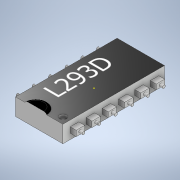
# Autodesk Inventor part: drive motor
Saved by Autodesk Inventor 2021 (Build 250183000, 183)
## iProperties
Created: 2021-07-29
Part Number: drive motor
Material: Generic
Document SubType Name: Modeling
Designer: Dell
Density: 1 g/cm^3
Appearance: Default
Author: Dell
Autodesk Inventor part; units mm, degrees
ref_plane "YZ Plane" through (0, 0, 0) normal (1, 0, 0) x (0, 1, 0)
ref_plane "XZ Plane" through (0, 0, 0) normal (0, 1, 0) x (-1, 0, 0)
ref_plane "XY Plane" through (0, 0, 0) normal (0, 0, 1) x (1, 0, 0)
sketch "Sketch1" plane through (0, 0, 0) normal (0, 1, 0) x (-1, 0, 0)
  line L0 (-9.2195, 27.5122) -> (18.7805, 27.5122)
  line L1 (18.7805, 27.5122) -> (18.7805, -32.4878)
  line L2 (18.7805, -32.4878) -> (-9.2195, -32.4878)
  line L3 (-9.2195, -32.4878) -> (-9.2195, 27.5122)
  point P0 (0, 0)
  dimension "d0" = 60
  dimension "d1" = 28
  constraints: 8 end point, 2 parallel, 1 horizontal, 1 perpendicular
  measures "d0" distance of L0.end L1.end
  measures "d1" distance of L0.start L0.end
extrude "Extrusion1" add sketch "Sketch1" along normal blind 10
sketch "Sketch2" plane through (9.2195, 0, 27.5122) normal (1, 0, 0) x (0, 0, -1)
  line L0 (60, 10) -> (0, 10) projected
  line L1 (60, 0) -> (0, 0) projected
  line L2 (4.3635, 6.5) -> (9.3635, 6.5)
  line L3 (9.3635, 6.5) -> (9.3635, 3.2102)
  line L4 (9.3635, 3.2102) -> (4.3635, 3.2102)
  line L5 (4.3635, 3.2102) -> (4.3635, 6.5)
  line L6 (13.6667, 6.5) -> (18.6667, 6.5)
  line L7 (18.6667, 6.5) -> (18.6667, 3.2102)
  line L8 (18.6667, 3.2102) -> (13.6667, 3.2102)
  line L9 (13.6667, 3.2102) -> (13.6667, 6.5)
  line L10 (23.1882, 6.5) -> (28.1882, 6.5)
  line L11 (28.1882, 6.5) -> (28.1882, 3.5)
  line L12 (28.1882, 3.5) -> (23.1882, 3.5)
  line L13 (23.1882, 3.5) -> (23.1882, 6.5)
  line L14 (32.8844, 6.5) -> (37.8844, 6.5)
  line L15 (37.8844, 6.5) -> (37.8844, 3.5)
  line L16 (37.8844, 3.5) -> (32.8844, 3.5)
  line L17 (32.8844, 3.5) -> (32.8844, 6.5)
  line L18 (42.406, 6.5) -> (47.406, 6.5)
  line L19 (47.406, 6.5) -> (47.406, 3.5)
  line L20 (47.406, 3.5) -> (42.406, 3.5)
  line L21 (42.406, 3.5) -> (42.406, 6.5)
  line L22 (51.5781, 6.5) -> (56.5781, 6.5)
  line L23 (56.5781, 6.5) -> (56.5781, 3.5)
  line L24 (56.5781, 3.5) -> (51.5781, 3.5)
  line L25 (51.5781, 3.5) -> (51.5781, 6.5)
  point P0 (27.5122, 0)
  point P1 (4.3635, 10)
  point P2 (4.3635, 0)
  point P3 (4.3635, 3.5)
  dimension "d4" = 10
  dimension "d5" = 3
  dimension "d6" = 3.5
  dimension "d7" = 3.5
  dimension "d8" = 5
  dimension "d9" = 5
  dimension "d10" = 5
  dimension "d11" = 5
  dimension "d12" = 5
  dimension "d13" = 5
  constraints: 48 end point, 12 parallel, 11 point on line, 6 horizontal, 6 perpendicular
  measures "d4" distance of point (4.364, 0) point (4.364, 10)
  measures "d5" distance of point (4.364, 3.5) L2.start
  measures "d6" distance of point (4.364, 0) point (4.364, 3.5)
  measures "d7" distance of point (4.364, 10) L2.start
  measures "d8" distance of L6.start L6.end
  measures "d9" distance of L2.start L2.end
  measures "d10" distance of L10.start L10.end
  measures "d11" distance of L14.start L14.end
  measures "d12" distance of L18.start L18.end
  measures "d13" distance of L22.start L22.end
extrude "Extrusion2" add sketch "Sketch2" along normal blind 3.5
sketch "Sketch3" plane through (-18.7805, 0, -32.4878) normal (-1, 0, 0) x (0, 0, 1)
  line L0 (3.4219, 6.5) -> (3.4219, 3.5) projected
  line L1 (8.4219, 3.5) -> (3.4219, 3.5) projected
  line L2 (3.4219, 6.5) -> (8.4219, 6.5)
  line L3 (8.4219, 6.5) -> (8.4219, 3.5)
  line L4 (8.4219, 3.5) -> (3.4219, 3.5)
  line L5 (3.4219, 3.5) -> (3.4219, 6.5)
  line L6 (12.594, 3.5) -> (12.594, 6.5) projected
  line L7 (17.594, 6.5) -> (17.594, 3.5) projected
  line L8 (12.594, 6.5) -> (17.594, 6.5)
  line L9 (17.594, 6.5) -> (17.594, 3.5)
  line L10 (17.594, 3.5) -> (12.594, 3.5)
  line L11 (12.594, 3.5) -> (12.594, 6.5)
  line L12 (22.1156, 6.5) -> (27.1156, 6.5) projected
  line L13 (27.1156, 6.5) -> (27.1156, 3.5) projected
  line L14 (22.1156, 6.5) -> (27.1156, 6.5)
  line L15 (27.1156, 6.5) -> (27.1156, 3.5)
  line L16 (27.1156, 3.5) -> (22.1156, 3.5)
  line L17 (22.1156, 3.5) -> (22.1156, 6.5)
  line L18 (31.8118, 6.5) -> (31.8118, 3.5) projected
  line L19 (36.8118, 6.5) -> (36.8118, 3.5) projected
  line L20 (31.8118, 6.5) -> (36.8118, 6.5)
  line L21 (36.8118, 6.5) -> (36.8118, 3.5)
  line L22 (36.8118, 3.5) -> (31.8118, 3.5)
  line L23 (31.8118, 3.5) -> (31.8118, 6.5)
  line L24 (41.3333, 3.2102) -> (41.3333, 6.5) projected
  line L25 (46.3333, 3.2102) -> (41.3333, 3.2102) projected
  line L26 (41.3333, 6.5) -> (46.3333, 6.5)
  line L27 (46.3333, 6.5) -> (46.3333, 3.2102)
  line L28 (46.3333, 3.2102) -> (41.3333, 3.2102)
  line L29 (41.3333, 3.2102) -> (41.3333, 6.5)
  line L30 (50.6365, 3.2102) -> (50.6365, 6.5) projected
  line L31 (55.6365, 3.2102) -> (50.6365, 3.2102) projected
  line L32 (50.6365, 6.5) -> (55.6365, 6.5)
  line L33 (55.6365, 6.5) -> (55.6365, 3.2102)
  line L34 (55.6365, 3.2102) -> (50.6365, 3.2102)
  line L35 (50.6365, 3.2102) -> (50.6365, 6.5)
  point P0 (32.4878, 0)
  constraints: 48 end point, 12 parallel, 6 horizontal, 6 perpendicular
extrude "Extrusion3" add sketch "Sketch3" along normal blind 3.5
sketch "Sketch4" plane through (-22.2805, 0, -32.4878) normal (-1, 0, 0) x (0, 0, 1)
  circle A0 centre (5.9219, 4.87) radius 0.85
  circle A1 centre (15.1045, 4.87) radius 0.85
  circle A2 centre (24.4513, 4.87) radius 0.85
  circle A3 centre (34.1912, 4.87) radius 0.85
  circle A4 centre (43.8874, 4.8551) radius 0.85
  circle A5 centre (53.3216, 4.8551) radius 0.85
  point P0 (32.4878, 0)
  dimension "d18" = 1.7
  dimension "d19" = 1.7
  dimension "d20" = 1.7
  dimension "d21" = 1.7
  dimension "d22" = 1.7
  dimension "d23" = 1.7
  constraints: 6 centre point
  measures "d18" diameter of A0
  measures "d19" diameter of A1
  measures "d20" diameter of A2
  measures "d21" diameter of A3
  measures "d22" diameter of A4
  measures "d23" diameter of A5
extrude "Extrusion4" add sketch "Sketch4" along normal blind 2
sketch "Sketch5" plane through (9.2195, 0, 27.5122) normal (1, 0, 0) x (0, 0, -1)
  circle A0 centre (6.6784, 4.8551) radius 0.85 projected
  circle A1 centre (6.6784, 4.8551) radius 0.85
  circle A2 centre (16.1126, 4.8551) radius 0.85 projected
  circle A3 centre (16.1126, 4.8551) radius 0.85
  circle A4 centre (25.8088, 4.87) radius 0.85 projected
  circle A5 centre (25.8088, 4.87) radius 0.85
  circle A6 centre (35.5487, 4.87) radius 0.85 projected
  circle A7 centre (35.5487, 4.87) radius 0.85
  circle A8 centre (44.8955, 4.87) radius 0.85 projected
  circle A9 centre (44.8955, 4.87) radius 0.85
  circle A10 centre (54.0781, 4.87) radius 0.85 projected
  circle A11 centre (54.0781, 4.87) radius 0.85
  point P0 (27.5122, 0)
  constraints: 6 centre point, 6 coincident
extrude "Extrusion5" add sketch "Sketch5" along normal blind 5 contours A2
sketch "Sketch6" plane through (12.7195, 0, 27.5122) normal (1, 0, 0) x (0, 0, -1)
  circle A0 centre (6.6784, 4.8551) radius 0.85 projected
  circle A1 centre (6.6784, 4.8551) radius 0.85
  circle A2 centre (25.8088, 4.87) radius 0.85 projected
  circle A3 centre (25.8088, 4.87) radius 0.85
  circle A4 centre (35.5487, 4.87) radius 0.85 projected
  circle A5 centre (35.5487, 4.87) radius 0.85
  circle A6 centre (44.8955, 4.87) radius 0.85 projected
  circle A7 centre (44.8955, 4.87) radius 0.85
  circle A8 centre (54.0781, 4.87) radius 0.85 projected
  circle A9 centre (54.0781, 4.87) radius 0.85
  circle A10 centre (16.1126, 4.87) radius 0.8352
  point P0 (27.5122, 0)
  constraints: 6 centre point, 5 coincident
extrude "Extrusion6" add sketch "Sketch6" along normal blind 2
sketch "Sketch7" plane through (0, 10, 0) normal (0, 1, 0) x (1, 0, 0)
  point P0 (0, 0)
  point P1 (5.5656, -23.7553)
hole "Hole1" at (5.5656, 10, 23.7553) direction (0, -1, 0) diameter 4 depth 2
sketch "Sketch8" plane through (0, 10, 0) normal (0, 1, 0) x (1, 0, 0)
  line L0 (-18.7805, -27.5122) -> (9.2195, -27.5122) projected
  arc A0 (-0.3099, -27.5122) -> (-13.121, -27.5122) centre (-6.7155, -27.5122) ccw
  point P0 (0, 0)
  constraints: 2 point on circle, 2 point on line, 1 centre point
extrude "Extrusion7" add sketch "Sketch8" along normal blind 1
fillet "Fillet1" radius 2 1 edges at (-6.7155, 11, 21.1067)
sketch "Sketch9" plane through (0, 10, 0) normal (0, 1, 0) x (1, 0, 0)
  line L0 (-15.1184, -15.9793) -> (-15.1184, 19.4933) construction
  line L1 (-15.1184, 19.4933) -> (-4.7205, 19.4933) construction
  line L2 (-4.7205, 19.4933) -> (-4.7205, -15.9793) construction
  line L3 (-4.7205, -15.9793) -> (-15.1184, -15.9793) construction
  point P0 (0, 0)
  constraints: 2 other
body "Solid1"
